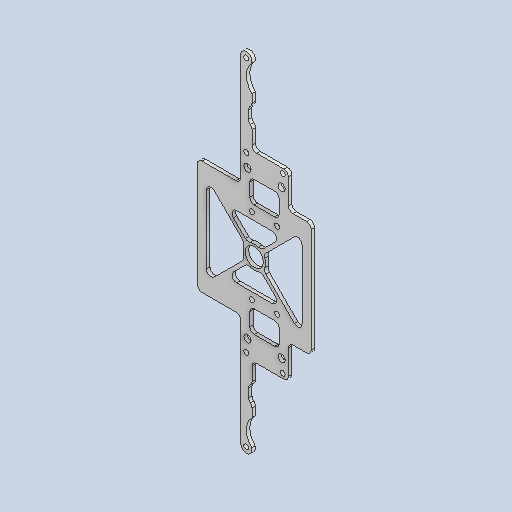
# Autodesk Inventor part: katasita
Saved by Autodesk Inventor 2025.1 (Build 291241000, 241)
## iProperties
Created: 2024-09-01
Part Number: katasita
Material: アルミニウム 2014-T4
Document SubType Name: Modeling
Designer: right
Density: 2.8 g/cm^3
Appearance: サテン
Mass: 8.59025 g
Surface Area: 54.0659 cm^2
Volume: 3.06795 cm^3
Author: right
Autodesk Inventor part; units mm, degrees
ref_plane "YZ Plane" through (0, 0, 0) normal (1, 0, 0) x (0, 1, 0)
ref_plane "XZ Plane" through (0, 0, 0) normal (0, 1, 0) x (-1, 0, 0)
ref_plane "XY Plane" through (0, 0, 0) normal (0, 0, 1) x (1, 0, 0)
sketch "スケッチ1" plane through (0, 0, 0) normal (0, 0, 1) x (1, 0, 0)
  circle A0 centre (20.9958, 34.5678) radius 1.1
  line L0 (20.9958, 34.5678) -> (9.9958, 34.5678) construction
  line L1 (9.9958, 34.5678) -> (9.9958, 1.0678) construction
  line L2 (9.9958, 1.0678) -> (20.9958, 1.0678) construction
  line L3 (20.9958, 1.0678) -> (20.9958, 34.5678) construction
  circle A1 centre (20.9958, 1.0678) radius 1.1
  circle A2 centre (9.9958, 34.5678) radius 1.1
  line L4 (25.9958, 57.8178) -> (4.9958, 57.8178)
  line L5 (4.9958, 57.8178) -> (4.9958, -22.1822)
  line L6 (4.9958, -22.1822) -> (25.9958, -22.1822)
  line L7 (25.9958, -22.1822) -> (25.9958, 57.8178)
  circle A3 centre (9.9958, 1.0678) radius 1.1
  point P0 (0, 0)
  point P1 (25.9958, 17.8178)
  point P2 (9.9958, 17.8178)
  point P3 (15.4958, -22.1822)
  point P4 (15.4958, 1.0678)
  dimension "d0" = 2.2
  dimension "d1" = 2.2
  dimension "d2" = 2.2
  dimension "d3" = 21
  dimension "d4" = 80
  dimension "d7" = 2.2
  dimension "d15" = 11
  dimension "d16" = 33.5
  constraints: 16 end point, 4 centre point, 4 midpoint, 4 parallel, 3 coincident, 2 horizontal, 2 perpendicular, 1 horizontal alignment, 1 vertical alignment
  measures "d0" diameter of A0
  measures "d1" diameter of A1
  measures "d2" diameter of A2
  measures "d3" distance of L5.end L6.end
  measures "d4" distance between parallel lines of L4 L6
  measures "d7" diameter of A3
  measures "d15" distance of L1.end L2.end
  measures "d16" distance of L0.end L1.end
extrude "押し出し1" add sketch "スケッチ1" along normal blind 1.5
sketch "スケッチ2" plane through (0, 0, 1.5) normal (0, 0, 1) x (1, 0, 0)
  circle A0 centre (7.4958, -20.1822) radius 1.1
  line L0 (4.9958, -22.1822) -> (25.9958, -22.1822) construction
  line L1 (15.4958, -22.1822) -> (15.4958, 57.8178) construction
  line L2 (25.9958, 57.8178) -> (4.9958, 57.8178) construction
  line L3 (4.9958, 57.8178) -> (4.9958, -22.1822) construction
  line L4 (4.9958, 17.8178) -> (25.9958, 17.8178) construction
  line L5 (25.9958, -22.1822) -> (25.9958, 57.8178) construction
  circle A1 centre (23.4958, -20.1822) radius 1.1
  circle A2 centre (7.4958, 55.8178) radius 1.1
  line L6 (25.9958, 57.8178) -> (25.9958, -22.1822) construction
  circle A3 centre (23.4958, 55.8178) radius 1.1
  point P0 (0, 0)
  dimension "d8" = 2.2
  dimension "d9" = 2.2
  dimension "d10" = 16
  dimension "d11" = 8
  dimension "d12" = 2
  constraints: 6 end point, 4 centre point, 4 midpoint, 4 symmetric about line, 1 horizontal alignment, 2 other
  measures "d8" diameter of A0
  measures "d9" diameter of A1
  measures "d10" distance of A0.centre A1.centre
  measures "d11" distance from line of L1 A1.centre
  measures "d12" distance from line of L0 A1.centre
extrude "押し出し2" cut sketch "スケッチ2" against normal through all
sketch "スケッチ3" plane through (0, 0, 1.5) normal (0, 0, 1) x (1, 0, 0)
  circle A0 centre (7.4958, 91.8178) radius 1.8 projected
  circle A1 centre (7.4958, 91.8178) radius 1.1
  circle A2 centre (7.4958, 91.8178) radius 2.5
  line L0 (25.9958, 57.8178) -> (4.9958, 57.8178) projected
  line L1 (4.9958, 57.8178) -> (4.9958, 91.8178)
  circle A3 centre (15.4958, 85.3178) radius 3 projected
  circle A4 centre (15.4958, 85.3178) radius 8 projected
  line L2 (9.9958, 91.8178) -> (9.9958, 57.8178)
  line L3 (25.9958, -22.1822) -> (25.9958, 57.8178) construction
  line L4 (25.9958, 17.8178) -> (4.9958, 17.8178) construction
  line L5 (4.9958, 57.8178) -> (4.9958, -22.1822) construction
  circle A5 centre (7.4958, -56.1822) radius 1.1
  circle A6 centre (7.4958, -56.1822) radius 2.5
  line L6 (4.9958, -22.1822) -> (4.9958, -56.1822)
  line L7 (9.9958, -56.1822) -> (9.9958, -22.1822)
  line L8 (4.9958, -22.1822) -> (25.9958, -22.1822) projected
  circle A7 centre (15.4958, -49.6822) radius 8 projected
  point P0 (0, 0)
  point P1 (4.9958, 91.5212)
  point P2 (4.9958, -55.8857)
  point P3 (9.855, -55.3551)
  point P4 (8.7883, -54.0423)
  point P5 (8.7883, 89.6778)
  point P6 (9.855, 90.9906)
  point P7 (9.9958, 79.5083)
  point P8 (9.9958, -43.8728)
  dimension "d17" = 2.2
  constraints: 10 end point, 6 symmetric about line, 4 centre point, 4 coincident, 4 point on circle, 3 point on line, 2 midpoint, 2 tangent, 2 vertical, 2 other
  measures "d17" diameter of A1
extrude "押し出し3" add sketch "スケッチ3" against normal up to surface (1.5 mm away) contours A0 | A2 A4 | A2 A4 L2 L0 L1 | A6 A7 | L6 L8 L7 A7 A6 picked at (5.6851, 93.1555) picked at (9.4943, -56.4694)
fillet "フィレット1" radius 2 4 edges at (9.9958, 57.8178, 0.75) (9.9958, -22.1822, 0.75) (25.9958, -22.1822, 0.75) (25.9958, 57.8178, 0.75)
sketch "スケッチ4" plane through (0, 0, 0) normal (0, 0, -1) x (-1, 0, 0)
  line L0 (-9.0671, -38.3608) -> (-12.9244, -38.3608) projected
  line L1 (-5.4958, -18.6822) -> (-5.4958, -57.6822) projected
  arc A0 (-5.4958, -18.6822) -> (-5.9958, -18.1822) centre (-5.9958, -18.6822) ccw projected
  line L2 (-24.9958, -18.1822) -> (-5.9958, -18.1822) projected
  arc A1 (-24.9958, -18.1822) -> (-25.4958, -18.6822) centre (-24.9958, -18.6822) ccw projected
  line L3 (-25.4958, -57.6822) -> (-25.4958, -18.6822) projected
  arc A2 (-25.4958, -57.6822) -> (-24.9958, -58.1822) centre (-24.9958, -57.6822) ccw projected
  line L4 (-5.9958, -58.1822) -> (-24.9958, -58.1822) projected
  arc A3 (-5.9958, -58.1822) -> (-5.4958, -57.6822) centre (-5.9958, -57.6822) ccw projected
  line L5 (-21.9244, -38.3608) -> (-21.9244, -32.0036) projected
  line L6 (-21.9244, -32.0036) -> (-18.0671, -32.0036) projected
  line L7 (-18.0671, -32.0036) -> (-18.0671, -38.3608) projected
  line L8 (-18.0671, -38.3608) -> (-21.9244, -38.3608) projected
  circle A4 centre (-15.4958, -30.7822) radius 1.1519 projected
  line L9 (-9.0671, -38.3608) -> (-12.9244, -38.3608) projected
  line L10 (-12.9244, -38.3608) -> (-12.9244, -32.0036) projected
  line L11 (-12.9244, -32.0036) -> (-9.0671, -32.0036) projected
  line L12 (-9.0671, -32.0036) -> (-9.0671, -38.3608) projected
  circle A5 centre (-23.4958, -56.1822) radius 1.8131 projected
  circle A6 centre (-7.4958, -56.1822) radius 1.8131 projected
  circle A7 centre (-23.4958, -20.1822) radius 1.8131 projected
  circle A8 centre (-7.4958, -20.1822) radius 1.8131 projected
  arc A9 (-21.7457, -49.6929) -> (-9.2458, -49.6822) centre (-15.4958, -49.6822) ccw projected
  arc A10 (-21.9958, -49.9322) -> (-21.746, -49.6929) centre (-21.9958, -49.6822) ccw projected
  line L13 (-21.9958, -49.9322) -> (-23.7458, -49.9322) projected
  arc A11 (-23.7458, -49.4322) -> (-23.7458, -49.9322) centre (-23.7458, -49.6822) ccw projected
  line L14 (-23.7458, -49.4322) -> (-21.9958, -49.4322) projected
  arc A12 (-21.7458, -49.6822) -> (-21.9958, -49.4322) centre (-21.9958, -49.6822) ccw projected
  arc A13 (-21.27, -47.2905) -> (-21.7458, -49.6822) centre (-15.4958, -49.6822) ccw projected
  arc A14 (-21.5966, -47.4258) -> (-21.27, -47.2905) centre (-21.501, -47.1948) ccw projected
  line L15 (-21.5966, -47.4258) -> (-23.2134, -46.7561) projected
  arc A15 (-23.0221, -46.2941) -> (-23.2134, -46.7561) centre (-23.1178, -46.5251) ccw projected
  line L16 (-23.0221, -46.2941) -> (-21.4053, -46.9638) projected
  arc A16 (-21.27, -47.2905) -> (-21.4053, -46.9638) centre (-21.501, -47.1948) ccw projected
  arc A17 (-19.9152, -45.2628) -> (-21.27, -47.2905) centre (-15.4958, -49.6822) ccw projected
  arc A18 (-20.2687, -45.2628) -> (-19.9152, -45.2628) centre (-20.0919, -45.086) ccw projected
  line L17 (-20.2687, -45.2628) -> (-21.5062, -44.0254) projected
  arc A19 (-21.1526, -43.6718) -> (-21.5062, -44.0254) centre (-21.3294, -43.8486) ccw projected
  line L18 (-21.1526, -43.6718) -> (-19.9152, -44.9093) projected
  arc A20 (-19.9152, -45.2628) -> (-19.9152, -44.9093) centre (-20.0919, -45.086) ccw projected
  arc A21 (-17.8875, -43.908) -> (-19.9152, -45.2628) centre (-15.4958, -49.6822) ccw projected
  arc A22 (-18.2142, -43.7727) -> (-17.8875, -43.908) centre (-17.9832, -43.677) ccw projected
  line L19 (-18.2142, -43.7727) -> (-18.8839, -42.1559) projected
  arc A23 (-18.4219, -41.9646) -> (-18.8839, -42.1559) centre (-18.6529, -42.0602) ccw projected
  line L20 (-18.4219, -41.9646) -> (-17.7522, -43.5813) projected
  arc A24 (-17.8875, -43.908) -> (-17.7522, -43.5813) centre (-17.9832, -43.677) ccw projected
  arc A25 (-15.4958, -43.4322) -> (-17.8875, -43.908) centre (-15.4958, -49.6822) ccw projected
  arc A26 (-15.7458, -43.1822) -> (-15.4958, -43.4322) centre (-15.4958, -43.1822) ccw projected
  line L21 (-15.7458, -43.1822) -> (-15.7458, -41.4322) projected
  arc A27 (-15.2458, -41.4322) -> (-15.7458, -41.4322) centre (-15.4958, -41.4322) ccw projected
  line L22 (-15.2458, -41.4322) -> (-15.2458, -43.1822) projected
  arc A28 (-15.4958, -43.4322) -> (-15.2458, -43.1822) centre (-15.4958, -43.1822) ccw projected
  arc A29 (-13.104, -43.908) -> (-15.4958, -43.4322) centre (-15.4958, -49.6822) ccw projected
  arc A30 (-13.2393, -43.5813) -> (-13.104, -43.908) centre (-13.0083, -43.677) ccw projected
  line L23 (-13.2393, -43.5813) -> (-12.5696, -41.9646) projected
  arc A31 (-12.1076, -42.1559) -> (-12.5696, -41.9646) centre (-12.3386, -42.0602) ccw projected
  line L24 (-12.1076, -42.1559) -> (-12.7773, -43.7727) projected
  arc A32 (-13.104, -43.908) -> (-12.7773, -43.7727) centre (-13.0083, -43.677) ccw projected
  arc A33 (-11.0763, -45.2628) -> (-13.104, -43.908) centre (-15.4958, -49.6822) ccw projected
  arc A34 (-11.0763, -44.9093) -> (-11.0763, -45.2628) centre (-10.8996, -45.086) ccw projected
  line L25 (-11.0763, -44.9093) -> (-9.8389, -43.6718) projected
  arc A35 (-9.4853, -44.0254) -> (-9.8389, -43.6718) centre (-9.6621, -43.8486) ccw projected
  line L26 (-9.4853, -44.0254) -> (-10.7228, -45.2628) projected
  arc A36 (-11.0763, -45.2628) -> (-10.7228, -45.2628) centre (-10.8996, -45.086) ccw projected
  arc A37 (-9.7215, -47.2905) -> (-11.0763, -45.2628) centre (-15.4958, -49.6822) ccw projected
  arc A38 (-9.5862, -46.9638) -> (-9.7215, -47.2905) centre (-9.4905, -47.1948) ccw projected
  line L27 (-9.5862, -46.9638) -> (-7.9694, -46.2941) projected
  arc A39 (-7.7781, -46.7561) -> (-7.9694, -46.2941) centre (-7.8737, -46.5251) ccw projected
  line L28 (-7.7781, -46.7561) -> (-9.3949, -47.4258) projected
  arc A40 (-9.7215, -47.2905) -> (-9.3949, -47.4258) centre (-9.4905, -47.1948) ccw projected
  arc A41 (-9.2458, -49.6822) -> (-9.7215, -47.2905) centre (-15.4958, -49.6822) ccw projected
  arc A42 (-8.9958, -49.4322) -> (-9.2458, -49.6822) centre (-8.9958, -49.6822) ccw projected
  line L29 (-8.9958, -49.4322) -> (-7.2458, -49.4322) projected
  arc A43 (-7.2458, -49.9322) -> (-7.2458, -49.4322) centre (-7.2458, -49.6822) ccw projected
  line L30 (-7.2458, -49.9322) -> (-8.9958, -49.9322) projected
  arc A44 (-9.2458, -49.6822) -> (-8.9958, -49.9322) centre (-8.9958, -49.6822) ccw projected
  line L31 (-25.4958, 54.3178) -> (-25.4958, 93.3178) projected
  arc A45 (-25.4958, 54.3178) -> (-24.9958, 53.8178) centre (-24.9958, 54.3178) ccw projected
  line L32 (-5.9958, 53.8178) -> (-24.9958, 53.8178) projected
  arc A46 (-5.9958, 53.8178) -> (-5.4958, 54.3178) centre (-5.9958, 54.3178) ccw projected
  line L33 (-5.4958, 93.3178) -> (-5.4958, 54.3178) projected
  arc A47 (-5.4958, 93.3178) -> (-5.9958, 93.8178) centre (-5.9958, 93.3178) ccw projected
  line L34 (-24.9958, 93.8178) -> (-5.9958, 93.8178) projected
  arc A48 (-24.9958, 93.8178) -> (-25.4958, 93.3178) centre (-24.9958, 93.3178) ccw projected
  line L35 (-9.0671, 73.9964) -> (-9.0671, 67.6392) projected
  line L36 (-9.0671, 67.6392) -> (-12.9244, 67.6392) projected
  line L37 (-12.9244, 67.6392) -> (-12.9244, 73.9964) projected
  line L38 (-12.9244, 73.9964) -> (-9.0671, 73.9964) projected
  circle A49 centre (-15.4958, 66.4178) radius 1.1519 projected
  line L39 (-21.9244, 73.9964) -> (-18.0671, 73.9964) projected
  line L40 (-18.0671, 73.9964) -> (-18.0671, 67.6392) projected
  line L41 (-18.0671, 67.6392) -> (-21.9244, 67.6392) projected
  line L42 (-21.9244, 67.6392) -> (-21.9244, 73.9964) projected
  circle A50 centre (-7.4958, 91.8178) radius 1.8131 projected
  circle A51 centre (-23.4958, 91.8178) radius 1.8131 projected
  circle A52 centre (-7.4958, 55.8178) radius 1.8131 projected
  circle A53 centre (-23.4958, 55.8178) radius 1.8131 projected
  arc A54 (-9.2458, 85.3285) -> (-21.7458, 85.3178) centre (-15.4958, 85.3178) ccw projected
  arc A55 (-8.9958, 85.5678) -> (-9.2455, 85.3285) centre (-8.9958, 85.3178) ccw projected
  line L43 (-8.9958, 85.5678) -> (-7.2458, 85.5678) projected
  arc A56 (-7.2458, 85.0678) -> (-7.2458, 85.5678) centre (-7.2458, 85.3178) ccw projected
  line L44 (-7.2458, 85.0678) -> (-8.9958, 85.0678) projected
  arc A57 (-9.2458, 85.3178) -> (-8.9958, 85.0678) centre (-8.9958, 85.3178) ccw projected
  arc A58 (-9.7215, 82.926) -> (-9.2458, 85.3178) centre (-15.4958, 85.3178) ccw projected
  arc A59 (-9.3949, 83.0613) -> (-9.7215, 82.926) centre (-9.4905, 82.8303) ccw projected
  line L45 (-9.3949, 83.0613) -> (-7.7781, 82.3916) projected
  arc A60 (-7.9694, 81.9297) -> (-7.7781, 82.3916) centre (-7.8737, 82.1606) ccw projected
  line L46 (-7.9694, 81.9297) -> (-9.5862, 82.5994) projected
  arc A61 (-9.7215, 82.926) -> (-9.5862, 82.5994) centre (-9.4905, 82.8303) ccw projected
  arc A62 (-11.0763, 80.8984) -> (-9.7215, 82.926) centre (-15.4958, 85.3178) ccw projected
  arc A63 (-10.7228, 80.8984) -> (-11.0763, 80.8984) centre (-10.8996, 80.7216) ccw projected
  line L47 (-10.7228, 80.8984) -> (-9.4853, 79.6609) projected
  arc A64 (-9.8389, 79.3074) -> (-9.4853, 79.6609) centre (-9.6621, 79.4841) ccw projected
  line L48 (-9.8389, 79.3074) -> (-11.0763, 80.5448) projected
  arc A65 (-11.0763, 80.8984) -> (-11.0763, 80.5448) centre (-10.8996, 80.7216) ccw projected
  arc A66 (-13.104, 79.5435) -> (-11.0763, 80.8984) centre (-15.4958, 85.3178) ccw projected
  arc A67 (-12.7773, 79.4082) -> (-13.104, 79.5435) centre (-13.0083, 79.3126) ccw projected
  line L49 (-12.7773, 79.4082) -> (-12.1076, 77.7914) projected
  arc A68 (-12.5696, 77.6001) -> (-12.1076, 77.7914) centre (-12.3386, 77.6958) ccw projected
  line L50 (-12.5696, 77.6001) -> (-13.2393, 79.2169) projected
  arc A69 (-13.104, 79.5435) -> (-13.2393, 79.2169) centre (-13.0083, 79.3126) ccw projected
  arc A70 (-15.4958, 79.0678) -> (-13.104, 79.5435) centre (-15.4958, 85.3178) ccw projected
  arc A71 (-15.2458, 78.8178) -> (-15.4958, 79.0678) centre (-15.4958, 78.8178) ccw projected
  line L51 (-15.2458, 78.8178) -> (-15.2458, 77.0678) projected
  arc A72 (-15.7458, 77.0678) -> (-15.2458, 77.0678) centre (-15.4958, 77.0678) ccw projected
  line L52 (-15.7458, 77.0678) -> (-15.7458, 78.8178) projected
  arc A73 (-15.4958, 79.0678) -> (-15.7458, 78.8178) centre (-15.4958, 78.8178) ccw projected
  arc A74 (-17.8875, 79.5435) -> (-15.4958, 79.0678) centre (-15.4958, 85.3178) ccw projected
  arc A75 (-17.7522, 79.2169) -> (-17.8875, 79.5435) centre (-17.9832, 79.3126) ccw projected
  line L53 (-17.7522, 79.2169) -> (-18.4219, 77.6001) projected
  arc A76 (-18.8839, 77.7914) -> (-18.4219, 77.6001) centre (-18.6529, 77.6958) ccw projected
  line L54 (-18.8839, 77.7914) -> (-18.2142, 79.4082) projected
  arc A77 (-17.8875, 79.5435) -> (-18.2142, 79.4082) centre (-17.9832, 79.3126) ccw projected
  arc A78 (-19.9152, 80.8984) -> (-17.8875, 79.5435) centre (-15.4958, 85.3178) ccw projected
  arc A79 (-19.9152, 80.5448) -> (-19.9152, 80.8984) centre (-20.0919, 80.7216) ccw projected
  line L55 (-19.9152, 80.5448) -> (-21.1526, 79.3074) projected
  arc A80 (-21.5062, 79.6609) -> (-21.1526, 79.3074) centre (-21.3294, 79.4841) ccw projected
  line L56 (-21.5062, 79.6609) -> (-20.2687, 80.8984) projected
  arc A81 (-19.9152, 80.8984) -> (-20.2687, 80.8984) centre (-20.0919, 80.7216) ccw projected
  arc A82 (-21.27, 82.926) -> (-19.9152, 80.8984) centre (-15.4958, 85.3178) ccw projected
  arc A83 (-21.4053, 82.5994) -> (-21.27, 82.926) centre (-21.501, 82.8303) ccw projected
  line L57 (-21.4053, 82.5994) -> (-23.0221, 81.9297) projected
  arc A84 (-23.2134, 82.3916) -> (-23.0221, 81.9297) centre (-23.1178, 82.1606) ccw projected
  line L58 (-23.2134, 82.3916) -> (-21.5966, 83.0613) projected
  arc A85 (-21.27, 82.926) -> (-21.5966, 83.0613) centre (-21.501, 82.8303) ccw projected
  arc A86 (-21.7458, 85.3178) -> (-21.27, 82.926) centre (-15.4958, 85.3178) ccw projected
  arc A87 (-21.9958, 85.0678) -> (-21.7458, 85.3178) centre (-21.9958, 85.3178) ccw projected
  line L59 (-21.9958, 85.0678) -> (-23.7458, 85.0678) projected
  arc A88 (-23.7458, 85.5678) -> (-23.7458, 85.0678) centre (-23.7458, 85.3178) ccw projected
  line L60 (-23.7458, 85.5678) -> (-21.9958, 85.5678) projected
  arc A89 (-21.7458, 85.3178) -> (-21.9958, 85.5678) centre (-21.9958, 85.3178) ccw projected
  line L61 (-12.9244, 73.9964) -> (-9.0671, 73.9964) projected
  line L62 (-13.5244, 74.5964) -> (-13.5244, 67.0392)
  line L63 (-13.5244, 67.0392) -> (-8.4671, 67.0392)
  line L64 (-8.4671, 67.0392) -> (-8.4671, 74.5964)
  line L65 (-13.5244, 74.5964) -> (-8.4671, 74.5964)
  line L66 (-8.4671, -38.9608) -> (-8.4671, -31.4036)
  line L67 (-8.4671, -31.4036) -> (-13.5244, -31.4036)
  line L68 (-13.5244, -31.4036) -> (-13.5244, -38.9608)
  line L69 (-8.4671, -38.9608) -> (-13.5244, -38.9608)
  point P0 (0, 0)
  dimension "d22" = 0.6
  dimension "d23" = 0.6
  dimension "d24" = 0.6
  dimension "d25" = 0.6
  constraints: 16 end point, 2 parallel, 4 other
  measures "d22" distance between parallel lines of L36 L63
  measures "d23" distance between parallel lines of L38 L65
  measures "d24" distance between parallel lines of L11 L67
  measures "d25" distance between parallel lines of L0 L69
extrude "押し出し4" cut sketch "スケッチ4" against normal through all contours L0 L10 L11 L12 | L35 L36 L37 L38 | L65 L64 L63 L62 | L69 L68 L67 L66
fillet "フィレット2" radius 2 8 edges at (9.9958, -31.4036, 0.75) (8.4671, -31.4036, 0.75) (8.4671, -38.9608, 0.75) (9.9958, -38.9608, 0.75) (9.9958, 67.0392, 0.75) (8.4671, 67.0392, 0.75) (8.4671, 74.5964, 0.75) (9.9958, 74.5964, 0.75)
sketch "スケッチ6" plane through (0, 0, 1.5) normal (0, 0, 1) x (1, 0, 0)
  circle A0 centre (-21.0042, 54.8178) radius 3 construction
  line L0 (-24.0042, 54.8178) -> (-24.0042, -19.1822) projected
  line L1 (1.9958, 57.8178) -> (-21.0042, 57.8178) projected
  circle A1 centre (1.9958, 54.8178) radius 3 construction
  line L2 (4.9958, 91.8178) -> (4.9958, -56.1822) projected
  line L3 (25.9958, -20.1822) -> (25.9958, 55.8178) construction
  line L4 (25.9958, 17.8178) -> (-24.0042, 17.8178) construction
  circle A2 centre (-21.0042, -19.1822) radius 3 construction
  circle A3 centre (1.9958, -19.1822) radius 3 construction
  circle A4 centre (1.9958, 54.8178) radius 1.6
  circle A5 centre (-21.0042, 54.8178) radius 1.6
  circle A6 centre (1.9958, -19.1822) radius 1.6
  circle A7 centre (-21.0042, -19.1822) radius 1.6
  point P0 (0, 0)
  point P1 (4.9958, 60.8178)
  dimension "d35" = 6
  dimension "d36" = 6
  dimension "d37" = 3.2
  dimension "d38" = 3.2
  constraints: 8 centre point, 4 symmetric about line, 3 tangent, 2 coincident, 2 end point, 2 midpoint, 1 horizontal alignment, 4 other
  measures "d35" diameter of A0
  measures "d36" diameter of A1
  measures "d37" diameter of A4
  measures "d38" diameter of A5
extrude "押し出し6" cut sketch "スケッチ6" against normal through all
sketch "スケッチ7" plane through (0, 0, 1.5) normal (0, 0, 1) x (1, 0, 0)
  line L0 (-14.0042, -7.1822) -> (35.9958, -7.1822)
  line L1 (35.9958, -7.1822) -> (35.9958, 42.8178)
  line L2 (35.9958, 42.8178) -> (-14.0042, 42.8178)
  line L3 (-14.0042, 42.8178) -> (-14.0042, -7.1822)
  line L4 (4.9958, 91.8178) -> (4.9958, -56.1822) projected
  line L5 (23.9958, 57.8178) -> (11.9958, 57.8178) projected
  line L6 (25.9958, -20.1822) -> (25.9958, -9.1822) projected
  line L7 (25.9958, -20.1822) -> (25.9958, 55.8178) projected
  point P0 (0, 0)
  point P1 (-14.0042, 17.8178)
  point P2 (4.9958, 17.8178)
  point P3 (10.9958, 42.8178)
  point P4 (17.9958, 57.8178)
  point P5 (25.9958, 42.8178)
  point P6 (25.9958, -7.1822)
  point P7 (4.9958, -7.1822)
  point P8 (4.9958, 42.8178)
  point P9 (25.9958, -14.6822)
  point P10 (25.9958, 42.8178)
  point P11 (25.9958, -7.1822)
  dimension "d41" = 50
  dimension "d42" = 50
  dimension "d46" = 10
  constraints: 8 end point, 5 midpoint, 2 parallel, 1 horizontal, 1 horizontal alignment, 1 perpendicular
  measures "d41" distance of L2.end L0.start
  measures "d42" distance of L1.end L2.end
  measures "d46" distance from line of point (25.996, -14.682) L1
extrude "押し出し7" add sketch "スケッチ7" against normal up to surface (1.5 mm away) contours L3 L2 L4 L0 | L7 L2 L1 L0
fillet "フィレット4" radius 2 4 edges at (25.9958, -7.1822, 0.75) (35.9958, -7.1822, 0.75) (35.9958, 42.8178, 0.75) (25.9958, 42.8178, 0.75)
fillet "フィレット5" radius 2 4 edges at (4.9958, -7.1822, 0.75) (-14.0042, -7.1822, 0.75) (-14.0042, 42.8178, 0.75) (4.9958, 42.8178, 0.75)
sketch "スケッチ8" plane through (0, 0, 1.5) normal (0, 0, 1) x (1, 0, 0)
  circle A0 centre (30.9958, 17.8178) radius 1.1 projected
  circle A1 centre (25.9958, 12.8178) radius 1.1 projected
  circle A2 centre (20.9958, 17.8178) radius 1.1 projected
  circle A3 centre (25.9958, 22.8178) radius 1.1 projected
  arc A4 (4.9958, -20.1822) -> (6.9958, -22.1822) centre (6.9958, -20.1822) ccw projected
  line L0 (6.9958, -22.1822) -> (23.9958, -22.1822) projected
  arc A5 (23.9958, -22.1822) -> (25.9958, -20.1822) centre (23.9958, -20.1822) ccw projected
  line L1 (25.9958, -20.1822) -> (25.9958, -9.1822) projected
  arc A6 (27.9958, -7.1822) -> (25.9958, -9.1822) centre (27.9958, -9.1822) ccw projected
  line L2 (27.9958, -7.1822) -> (33.9958, -7.1822) projected
  arc A7 (33.9958, -7.1822) -> (35.9958, -5.1822) centre (33.9958, -5.1822) ccw projected
  line L3 (35.9958, -5.1822) -> (35.9958, 40.8178) projected
  arc A8 (35.9958, 40.8178) -> (33.9958, 42.8178) centre (33.9958, 40.8178) ccw projected
  line L4 (33.9958, 42.8178) -> (27.9958, 42.8178) projected
  arc A9 (25.9958, 44.8178) -> (27.9958, 42.8178) centre (27.9958, 44.8178) ccw projected
  line L5 (25.9958, 44.8178) -> (25.9958, 55.8178) projected
  arc A10 (25.9958, 55.8178) -> (23.9958, 57.8178) centre (23.9958, 55.8178) ccw projected
  line L6 (23.9958, 57.8178) -> (6.9958, 57.8178) projected
  arc A11 (6.9958, 57.8178) -> (4.9958, 55.8178) centre (6.9958, 55.8178) ccw projected
  line L7 (4.9958, 55.8178) -> (4.9958, 44.8178) projected
  arc A12 (2.9958, 42.8178) -> (4.9958, 44.8178) centre (2.9958, 44.8178) ccw projected
  line L8 (2.9958, 42.8178) -> (-12.0042, 42.8178) projected
  arc A13 (-12.0042, 42.8178) -> (-14.0042, 40.8178) centre (-12.0042, 40.8178) ccw projected
  line L9 (-14.0042, 40.8178) -> (-14.0042, -5.1822) projected
  arc A14 (-14.0042, -5.1822) -> (-12.0042, -7.1822) centre (-12.0042, -5.1822) ccw projected
  line L10 (-12.0042, -7.1822) -> (2.9958, -7.1822) projected
  arc A15 (4.9958, -9.1822) -> (2.9958, -7.1822) centre (2.9958, -9.1822) ccw projected
  line L11 (4.9958, -9.1822) -> (4.9958, -20.1822) projected
  circle A16 centre (7.4958, 55.8178) radius 1.1 projected
  circle A17 centre (7.4958, -20.1822) radius 1.1 projected
  circle A18 centre (23.4958, -20.1822) radius 1.1 projected
  circle A19 centre (23.4958, 55.8178) radius 1.1 projected
  circle A20 centre (22.9958, -14.6822) radius 3
  line L12 (25.9958, -20.1822) -> (25.9958, -9.1822) projected
  line L13 (5.9958, -17.6822) -> (24.9958, -17.6822) projected
  circle A21 centre (22.9958, -14.6822) radius 1.6
  line L14 (-14.0042, 17.8178) -> (35.9958, 17.8178) construction
  line L15 (15.4958, -22.1822) -> (15.4958, 57.8178) construction
  circle A22 centre (7.9958, -14.6822) radius 3
  circle A23 centre (7.9958, -14.6822) radius 1.6
  line L16 (44.9958, 17.8178) -> (-5.0042, 17.8178) construction
  line L17 (25.9958, 55.8178) -> (25.9958, 44.8178)
  line L18 (4.9958, 44.8178) -> (4.9958, 55.8178)
  circle A24 centre (22.9958, 50.3178) radius 3
  line L19 (25.9958, 55.8178) -> (25.9958, 44.8178)
  circle A25 centre (22.9958, 50.3178) radius 1.6
  line L20 (15.4958, 57.8178) -> (15.4958, -22.1822) construction
  circle A26 centre (7.9958, 50.3178) radius 3
  circle A27 centre (7.9958, 50.3178) radius 1.6
  circle A28 centre (7.9958, 50.3178) radius 1.6 projected
  circle A29 centre (22.9958, -14.6822) radius 1.6 projected
  circle A30 centre (22.9958, 50.3178) radius 1.6 projected
  circle A31 centre (7.9958, -14.6822) radius 1.6 projected
  circle A32 centre (25.9958, 17.8178) radius 3 projected
  line L21 (32.9958, 33.5751) -> (32.9958, 28.7265) projected
  arc A33 (30.1624, 26.9084) -> (32.9958, 28.7265) centre (30.9958, 28.7265) ccw projected
  arc A34 (30.1624, 26.9084) -> (26.9825, 27.769) centre (25.9958, 17.8178) ccw projected
  arc A35 (25.7656, 31.1734) -> (26.9825, 27.769) centre (27.1798, 29.7592) ccw projected
  line L22 (25.7656, 31.1734) -> (29.5815, 34.9893) projected
  arc A36 (32.9958, 33.5751) -> (29.5815, 34.9893) centre (30.9958, 33.5751) ccw projected
  circle A37 centre (10.9958, 17.8178) radius 4 projected
  line L23 (7.2307, 22.997) -> (-6.1758, 36.4036) projected
  arc A38 (-4.7616, 39.8178) -> (-6.1758, 36.4036) centre (-4.7616, 37.8178) ccw projected
  line L24 (-4.7616, 39.8178) -> (3.4958, 39.8178) projected
  arc A39 (28.1673, 36.4036) -> (26.7531, 39.8178) centre (26.7531, 37.8178) ccw projected
  line L25 (28.1673, 36.4036) -> (14.7608, 22.997) projected
  arc A40 (12.6749, 22.5274) -> (14.7608, 22.997) centre (13.3466, 24.4112) ccw projected
  arc A41 (12.6749, 22.5274) -> (9.3166, 22.5274) centre (10.9958, 17.8178) ccw projected
  arc A42 (7.2307, 22.997) -> (9.3166, 22.5274) centre (8.6449, 24.4112) ccw projected
  arc A43 (26.9825, 7.8666) -> (30.1624, 8.7272) centre (25.9958, 17.8178) ccw projected
  arc A44 (32.9958, 6.9091) -> (30.1624, 8.7272) centre (30.9958, 6.9091) ccw projected
  line L26 (32.9958, 6.9091) -> (32.9958, 2.0604) projected
  arc A45 (29.5815, 0.6462) -> (32.9958, 2.0604) centre (30.9958, 2.0604) ccw projected
  line L27 (29.5815, 0.6462) -> (25.7656, 4.4621) projected
  arc A46 (26.9825, 7.8666) -> (25.7656, 4.4621) centre (27.1798, 5.8763) ccw projected
  line L28 (14.7608, 12.6385) -> (28.1673, -0.768) projected
  arc A47 (26.7531, -4.1822) -> (28.1673, -0.768) centre (26.7531, -2.1822) ccw projected
  line L29 (26.7531, -4.1822) -> (14.4958, -4.1822) projected
  arc A48 (-6.1758, -0.768) -> (-4.7616, -4.1822) centre (-4.7616, -2.1822) ccw projected
  line L30 (-6.1758, -0.768) -> (7.2307, 12.6385) projected
  arc A49 (9.3166, 13.1082) -> (7.2307, 12.6385) centre (8.6449, 11.2243) ccw projected
  arc A50 (9.3166, 13.1082) -> (12.6749, 13.1082) centre (10.9958, 17.8178) ccw projected
  arc A51 (14.7608, 12.6385) -> (12.6749, 13.1082) centre (13.3466, 11.2243) ccw projected
  line L31 (-7.59, 34.9893) -> (5.8165, 21.5828) projected
  arc A52 (6.2861, 19.4969) -> (5.8165, 21.5828) centre (4.4023, 20.1686) ccw projected
  arc A53 (6.2861, 19.4969) -> (6.2861, 16.1386) centre (10.9958, 17.8178) ccw projected
  arc A54 (5.8165, 14.0527) -> (6.2861, 16.1386) centre (4.4023, 15.467) ccw projected
  line L32 (5.8165, 14.0527) -> (-7.59, 0.6462) projected
  arc A55 (-11.0042, 2.0604) -> (-7.59, 0.6462) centre (-9.0042, 2.0604) ccw projected
  line L33 (-11.0042, 2.0604) -> (-11.0042, 33.5751) projected
  arc A56 (-7.59, 34.9893) -> (-11.0042, 33.5751) centre (-9.0042, 33.5751) ccw projected
  line L34 (19.9958, -9.1822) -> (19.9958, -17.1822) projected
  arc A57 (17.9958, -19.1822) -> (19.9958, -17.1822) centre (17.9958, -17.1822) ccw projected
  line L35 (17.9958, -19.1822) -> (12.9958, -19.1822) projected
  arc A58 (10.9958, -17.1822) -> (12.9958, -19.1822) centre (12.9958, -17.1822) ccw projected
  line L36 (10.9958, -17.1822) -> (10.9958, -9.1822) projected
  arc A59 (12.9958, -7.1822) -> (10.9958, -9.1822) centre (12.9958, -9.1822) ccw projected
  line L37 (12.9958, -7.1822) -> (17.9958, -7.1822) projected
  arc A60 (19.9958, -9.1822) -> (17.9958, -7.1822) centre (17.9958, -9.1822) ccw projected
  line L38 (12.9958, 54.8178) -> (17.9958, 54.8178) projected
  arc A61 (19.9958, 52.8178) -> (17.9958, 54.8178) centre (17.9958, 52.8178) ccw projected
  line L39 (19.9958, 52.8178) -> (19.9958, 44.8178) projected
  arc A62 (17.9958, 42.8178) -> (19.9958, 44.8178) centre (17.9958, 44.8178) ccw projected
  line L40 (17.9958, 42.8178) -> (12.9958, 42.8178) projected
  arc A63 (10.9958, 44.8178) -> (12.9958, 42.8178) centre (12.9958, 44.8178) ccw projected
  line L41 (10.9958, 44.8178) -> (10.9958, 52.8178) projected
  arc A64 (12.9958, 54.8178) -> (10.9958, 52.8178) centre (12.9958, 52.8178) ccw projected
  circle A65 centre (8.9958, -0.6822) radius 1.6 projected
  circle A66 centre (8.9958, 36.3178) radius 1.6 projected
  arc A67 (5.4958, 37.8178) -> (3.4958, 39.8178) centre (3.4958, 37.8178) ccw projected
  line L42 (5.4958, 37.8178) -> (5.4958, 36.3178) projected
  arc A68 (5.4958, 36.3178) -> (12.4958, 36.3178) centre (8.9958, 36.3178) ccw projected
  line L43 (12.4958, 36.3178) -> (12.4958, 37.8178) projected
  arc A69 (14.4958, 39.8178) -> (12.4958, 37.8178) centre (14.4958, 37.8178) ccw projected
  line L44 (14.4958, 39.8178) -> (26.7531, 39.8178) projected
  arc A70 (12.4958, -2.1822) -> (14.4958, -4.1822) centre (14.4958, -2.1822) ccw projected
  line L45 (12.4958, -2.1822) -> (12.4958, -0.6822) projected
  arc A71 (12.4958, -0.6822) -> (5.4958, -0.6822) centre (8.9958, -0.6822) ccw projected
  line L46 (5.4958, -0.6822) -> (5.4958, -2.1822) projected
  arc A72 (3.4958, -4.1822) -> (5.4958, -2.1822) centre (3.4958, -2.1822) ccw projected
  line L47 (3.4958, -4.1822) -> (-4.7616, -4.1822) projected
  point P0 (0, 0)
  dimension "d48" = 6
  dimension "d49" = 3.2
  constraints: 14 end point, 10 symmetric about line, 8 centre point, 4 coincident, 4 midpoint, 2 tangent, 6 other
  measures "d48" diameter of A20
  measures "d49" diameter of A21
extrude "押し出し8" cut sketch "スケッチ8" against normal through all contours A21 | A23 | A25 | A27
sketch "スケッチ9" plane through (0, 0, 1.5) normal (0, 0, 1) x (1, 0, 0)
  circle A0 centre (7.9958, 50.3178) radius 1.6 projected
  circle A1 centre (22.9958, -14.6822) radius 1.6 projected
  circle A2 centre (22.9958, 50.3178) radius 1.6 projected
  circle A3 centre (7.9958, -14.6822) radius 1.6 projected
  arc A4 (-12.0042, 42.8178) -> (-14.0042, 40.8178) centre (-12.0042, 40.8178) ccw projected
  line L0 (-14.0042, 40.8178) -> (-14.0042, -5.1822) projected
  arc A5 (-14.0042, -5.1822) -> (-12.0042, -7.1822) centre (-12.0042, -5.1822) ccw projected
  line L1 (-12.0042, -7.1822) -> (2.9958, -7.1822) projected
  arc A6 (4.9958, -9.1822) -> (2.9958, -7.1822) centre (2.9958, -9.1822) ccw projected
  line L2 (4.9958, -9.1822) -> (4.9958, -56.1822) projected
  arc A7 (4.9958, -56.1822) -> (9.855, -55.3551) centre (7.4958, -56.1822) ccw projected
  arc A8 (9.9958, -43.8728) -> (9.855, -55.3551) centre (15.4958, -49.6822) ccw projected
  line L3 (9.9958, -43.8728) -> (9.9958, -40.1624) projected
  arc A9 (9.9958, -40.1624) -> (9.2314, -38.5898) centre (7.9958, -40.1624) ccw projected
  arc A10 (8.4671, -37.0172) -> (9.2314, -38.5898) centre (10.4671, -37.0172) ccw projected
  line L4 (8.4671, -37.0172) -> (8.4671, -33.3473) projected
  arc A11 (9.2314, -31.7747) -> (8.4671, -33.3473) centre (10.4671, -33.3473) ccw projected
  arc A12 (9.2314, -31.7747) -> (9.9958, -30.2021) centre (7.9958, -30.2021) ccw projected
  line L5 (9.9958, -30.2021) -> (9.9958, -24.1822) projected
  arc A13 (11.9958, -22.1822) -> (9.9958, -24.1822) centre (11.9958, -24.1822) ccw projected
  line L6 (11.9958, -22.1822) -> (23.9958, -22.1822) projected
  arc A14 (23.9958, -22.1822) -> (25.9958, -20.1822) centre (23.9958, -20.1822) ccw projected
  line L7 (25.9958, -20.1822) -> (25.9958, -9.1822) projected
  arc A15 (27.9958, -7.1822) -> (25.9958, -9.1822) centre (27.9958, -9.1822) ccw projected
  line L8 (27.9958, -7.1822) -> (33.9958, -7.1822) projected
  arc A16 (33.9958, -7.1822) -> (35.9958, -5.1822) centre (33.9958, -5.1822) ccw projected
  line L9 (35.9958, -5.1822) -> (35.9958, 40.8178) projected
  arc A17 (35.9958, 40.8178) -> (33.9958, 42.8178) centre (33.9958, 40.8178) ccw projected
  line L10 (33.9958, 42.8178) -> (27.9958, 42.8178) projected
  arc A18 (25.9958, 44.8178) -> (27.9958, 42.8178) centre (27.9958, 44.8178) ccw projected
  line L11 (25.9958, 44.8178) -> (25.9958, 55.8178) projected
  arc A19 (25.9958, 55.8178) -> (23.9958, 57.8178) centre (23.9958, 55.8178) ccw projected
  line L12 (23.9958, 57.8178) -> (11.9958, 57.8178) projected
  arc A20 (9.9958, 59.8178) -> (11.9958, 57.8178) centre (11.9958, 59.8178) ccw projected
  line L13 (9.9958, 59.8178) -> (9.9958, 65.8376) projected
  arc A21 (9.9958, 65.8376) -> (9.2314, 67.4102) centre (7.9958, 65.8376) ccw projected
  arc A22 (8.4671, 68.9828) -> (9.2314, 67.4102) centre (10.4671, 68.9828) ccw projected
  line L14 (8.4671, 68.9828) -> (8.4671, 72.6527) projected
  arc A23 (9.2314, 74.2253) -> (8.4671, 72.6527) centre (10.4671, 72.6527) ccw projected
  arc A24 (9.2314, 74.2253) -> (9.9958, 75.7979) centre (7.9958, 75.7979) ccw projected
  line L15 (9.9958, 75.7979) -> (9.9958, 79.5083) projected
  arc A25 (9.855, 90.9906) -> (9.9958, 79.5083) centre (15.4958, 85.3178) ccw projected
  arc A26 (9.855, 90.9906) -> (4.9958, 91.8178) centre (7.4958, 91.8178) ccw projected
  line L16 (4.9958, 91.8178) -> (4.9958, 44.8178) projected
  arc A27 (2.9958, 42.8178) -> (4.9958, 44.8178) centre (2.9958, 44.8178) ccw projected
  line L17 (2.9958, 42.8178) -> (-12.0042, 42.8178) projected
  circle A28 centre (7.4958, -56.1822) radius 1.1 projected
  circle A29 centre (7.4958, 91.8178) radius 1.1 projected
  circle A30 centre (7.4958, -20.1822) radius 1.1 projected
  circle A31 centre (23.4958, 55.8178) radius 1.1 projected
  circle A32 centre (23.4958, -20.1822) radius 1.1 projected
  circle A33 centre (7.4958, 55.8178) radius 1.1 projected
  circle A34 centre (20.9958, 1.0678) radius 1.1 projected
  circle A35 centre (9.9958, 34.5678) radius 1.1 projected
  circle A36 centre (9.9958, 1.0678) radius 1.1 projected
  circle A37 centre (20.9958, 34.5678) radius 1.1 projected
  line L18 (-10.0042, 38.8178) -> (31.9958, 38.8178)
  line L19 (31.9958, 38.8178) -> (31.9958, -3.1822)
  line L20 (31.9958, -3.1822) -> (-10.0042, -3.1822)
  line L21 (-10.0042, -3.1822) -> (-10.0042, 38.8178)
  line L22 (-13.8382, 38.8178) -> (23.9958, 38.8178)
  line L23 (23.9958, 38.8178) -> (23.9958, 31.5678)
  line L24 (23.9958, 31.5678) -> (-13.8382, 31.5678)
  line L25 (-13.8382, 31.5678) -> (-13.8382, 38.8178)
  circle A38 centre (9.9958, 34.5678) radius 3
  circle A39 centre (20.9958, 34.5678) radius 3
  line L26 (31.9958, 17.8178) -> (-10.0042, 17.8178) construction
  line L27 (23.9958, -3.1822) -> (23.9958, 4.0678)
  line L28 (23.9958, 4.0678) -> (-13.8382, 4.0678)
  line L29 (-13.8382, 4.0678) -> (-13.8382, -3.1822)
  line L30 (31.9958, 38.8178) -> (-10.0042, -3.1822) construction
  line L31 (31.9958, -3.1822) -> (-10.0042, 38.8178) construction
  circle A40 centre (10.9958, 17.8178) radius 4
  circle A41 centre (10.9958, 17.8178) radius 5
  line L32 (-8.8729, -3.1822) -> (31.9958, 37.6864)
  line L33 (-10.0042, -2.0509) -> (30.8644, 38.8178)
  line L34 (-8.8729, 38.8178) -> (31.9958, -2.0509)
  line L35 (-10.0042, 37.6864) -> (30.8644, -3.1822)
  point P0 (0, 0)
  point P1 (23.9958, 31.9491)
  point P2 (30.8644, 38.8178)
  point P3 (30.8644, -3.1822)
  point P4 (23.9958, 3.6864)
  point P5 (23.6144, 4.0678)
  point P6 (13.9201, 13.7621)
  point P7 (8.0715, 13.7621)
  point P8 (6.9958, -3.1822)
  point P9 (15.0514, 14.8935)
  point P10 (31.9958, -2.0509)
  point P11 (15.0514, 20.7421)
  point P12 (8.0715, 21.8734)
  point P13 (13.9201, 21.8734)
  point P14 (23.6144, 31.5678)
  point P15 (6.9401, 20.7421)
  point P16 (-10.0042, 37.6864)
  point P17 (-10.0042, -2.0509)
  point P18 (6.9401, 14.8935)
  point P19 (-1.6229, 4.0678)
  point P20 (10.9958, 16.6864)
  point P21 (-10.0042, 4.0678)
  point P22 (-10.0042, 31.5678)
  point P23 (10.9958, 18.9491)
  point P24 (-1.6229, 31.5678)
  point P25 (-3.8856, 4.0678)
  point P26 (12.1271, 17.8178)
  point P27 (9.8644, 17.8178)
  dimension "d52" = 4
  dimension "d53" = 4
  dimension "d54" = 4
  dimension "d55" = 4
  dimension "d56" = 6
  dimension "d57" = 6
  dimension "d58" = 8
  dimension "d59" = 10
  dimension "d60" = 0.8
  constraints: 36 end point, 10 symmetric about line, 5 parallel, 4 centre point, 3 coincident, 3 midpoint, 3 point on line, 2 horizontal, 2 perpendicular, 2 tangent
  measures "d52" distance between parallel lines of L17 L18
  measures "d53" distance between parallel lines of L0 L21
  measures "d54" distance between parallel lines of L9 L19
  measures "d55" distance between parallel lines of L1 L20
  measures "d56" diameter of A38
  measures "d57" diameter of A39
  measures "d58" diameter of A40
  measures "d59" diameter of A41
  measures "d60" distance between parallel lines of L33 L30
extrude "押し出し9" cut sketch "スケッチ9" against normal through all contours A34 | A35 | A36 | A37 | L35 L24 L21 | L24 L33 A41 L34 | L24 L35 A41 L33 L28 L21 | L28 L33 L21 | L34 L33 L35 A40 | A40 L33 L34 | L35 L33 A40 | L19 L34 A41 L32 | A40 L32 L34 L33 | L34 L32 L35 L33 | L32 A41 L35 L28 | L33 L35 L32 A40 | A40 L34 L32 | L34 A40 L35 L32 | L32 L35 A40
fillet "フィレット6" radius 2 16 edges at (31.9958, 37.6864, 0.75) (31.9958, -2.0509, 0.75) (23.6144, 4.0678, 0.75) (13.9201, 13.7621, 0.75) (15.0514, 14.8935, 0.75) (15.0514, 20.7421, 0.75) (13.9201, 21.8734, 0.75) (23.6144, 31.5678, 0.75) (8.0715, 21.8734, 0.75) (6.9401, 20.7421, 0.75) (-10.0042, 37.6864, 0.75) (8.0715, 13.7621, 0.75) (6.9401, 14.8935, 0.75) (-1.6229, 4.0678, 0.75) (-10.0042, -2.0509, 0.75) (-1.6229, 31.5678, 0.75)
sketch "スケッチ10" plane through (0, 0, 1.5) normal (0, 0, 1) x (1, 0, 0)
  line L0 (8.9958, -11.6822) -> (21.9958, -11.6822)
  line L1 (21.9958, -11.6822) -> (21.9958, -1.9322)
  line L2 (21.9958, -1.9322) -> (8.9958, -1.9322)
  line L3 (8.9958, -1.9322) -> (8.9958, -11.6822)
  circle A0 centre (9.9958, 1.0678) radius 1.1 projected
  circle A1 centre (9.9958, 1.0678) radius 3
  line L4 (6.9958, 2.0678) -> (6.9958, -1.1822) projected
  circle A2 centre (7.9958, -14.6822) radius 1.6 projected
  circle A3 centre (7.9958, -14.6822) radius 3
  line L5 (4.9958, -9.1822) -> (4.9958, -56.1822) projected
  line L6 (25.9958, -20.1822) -> (25.9958, -9.1822) projected
  line L7 (-14.0042, 40.8178) -> (-14.0042, -5.1822) construction
  circle A4 centre (10.9958, 17.8178) radius 4 construction
  line L8 (-14.0042, 17.8178) -> (10.9958, 17.8178) construction
  line L9 (8.9958, 47.3178) -> (21.9958, 47.3178)
  line L10 (21.9958, 47.3178) -> (21.9958, 37.5678)
  line L11 (21.9958, 37.5678) -> (8.9958, 37.5678)
  line L12 (8.9958, 37.5678) -> (8.9958, 47.3178)
  point P0 (0, 0)
  point P1 (4.9958, 44.8178)
  point P2 (25.9958, 44.8178)
  dimension "d64" = 4
  dimension "d65" = 4
  constraints: 18 end point, 6 symmetric about line, 4 tangent, 2 centre point, 2 coincident, 2 horizontal, 2 parallel, 1 midpoint, 1 perpendicular
  measures "d64" distance between parallel lines of L5 L3
  measures "d65" distance between parallel lines of L6 L1
extrude "押し出し10" cut sketch "スケッチ10" against normal through all contours L3 L2 L1 L0 | L9 L10 L11 L12
fillet "フィレット7" radius 2 8 edges at (21.9958, -11.6822, 0.75) (21.9958, -1.9322, 0.75) (8.9958, -1.9322, 0.75) (8.9958, -11.6822, 0.75) (8.9958, 47.3178, 0.75) (21.9958, 37.5678, 0.75) (8.9958, 37.5678, 0.75) (21.9958, 47.3178, 0.75)
equation "\"d22\" = d23"
equation "\"d24\" = d25"
equation "\"d25\" = d22"
